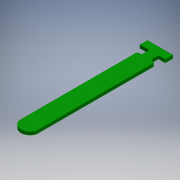
# Autodesk Inventor part: bracelet
Saved by Autodesk Inventor 2017 (Build 210142000, 142)
## iProperties
Part Number: bracelet
Material: Caoutchouc
Document SubType Name: Modeling
Designer: starl
Density: 0.93 g/cm^3
Appearance: Caoutchouc - Noir
Author: starl
Autodesk Inventor part; units mm, degrees
ref_plane "YZ Plane" through (0, 0, 0) normal (1, 0, 0) x (0, 1, 0)
ref_plane "XZ Plane" through (0, 0, 0) normal (0, 1, 0) x (-1, 0, 0)
ref_plane "XY Plane" through (0, 0, 0) normal (0, 0, 1) x (1, 0, 0)
sketch "Esquisse4" plane through (0, 0, 0) normal (0, 0, 1) x (1, 0, 0)
  line L0 (0, 0) -> (9, 0)
  line L1 (9, 0) -> (9, -7.36)
  line L2 (9, -7.36) -> (13, -7.36)
  line L3 (13, -7.36) -> (13, -122.36)
  line L4 (13, -122.36) -> (-4, -122.36)
  line L5 (-4, -122.36) -> (-4, -7.36)
  line L6 (-4, -7.36) -> (0, -7.36)
  line L7 (0, -7.36) -> (0, 0)
  arc A0 (-4, -122.36) -> (13, -122.36) centre (4.5, -120.3919) ccw
  line L8 (-9.0237, 0) -> (15.6194, 0)
  line L9 (15.6194, 0) -> (15.6194, 7.3414)
  line L10 (15.6194, 7.3414) -> (-9.0237, 7.3414)
  line L11 (-9.0237, 7.3414) -> (-9.0237, 0)
  dimension "d8" = 4
  dimension "d9" = 4
  dimension "d10" = 9
  dimension "d11" = 115
  dimension "d12" = 24.6431
  constraints: 24 end point, 7 perpendicular, 2 horizontal, 2 parallel, 2 point on circle, 2 point on line, 1 centre point
  measures "d8" distance of L1.end L2.end
  measures "d9" distance of L5.end L6.end
  measures "d10" distance between parallel lines of L1 L7
  measures "d11" distance of L2.end L3.end
  measures "d12" distance of L9.end L10.end
extrude "Extrusion1" add sketch "Esquisse4" along normal blind 3
fillet "Congé1" radius 2 2 edges at (13, -7.36, 1.5) (-4, -7.36, 1.5)
hole "Perçage1" at (4.6143, -119.075, 0) direction (0, 0, 1) diameter 0.5 end through all
pattern_linear "Réseau rectangulaire1" count 10 spacing 10 along (0, 1, 0) of "Perçage1"
sketch "Esquisse5" plane through (0, 0, 0) normal (0, 0, -1) x (-1, 0, 0)
  point P0 (0, 0)
